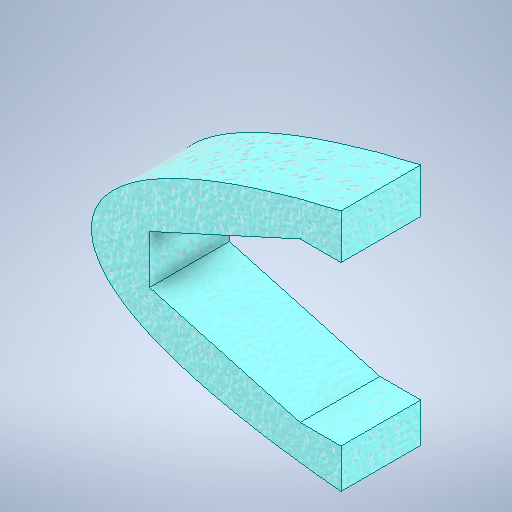
# Autodesk Inventor part: 2414 basic aerofoil
Saved by Autodesk Inventor 2025.1 (Build 291241000, 241)
## iProperties
Created: 2024-11-04
Part Number: 2414 basic aerofoil
Material: Polyurethane Foam
Document SubType Name: Modeling
Designer: johan
Density: 0.032 g/cm^3
Appearance: Coarse Textured - Umber
Author: johan
Autodesk Inventor part; units mm, degrees
ref_plane "YZ Plane" through (0, 0, 0) normal (1, 0, 0) x (0, 1, 0)
ref_plane "XZ Plane" through (0, 0, 0) normal (0, 1, 0) x (-1, 0, 0)
ref_plane "XY Plane" through (0, 0, 0) normal (0, 0, 1) x (1, 0, 0)
sketch "Sketch2" plane through (0, 0, 0) normal (0, 0, 1) x (1, 0, 0)
  spline S0 degree 5 poles (319.65, 0.0573) (319.6503, 0.0612) (319.6024, 0.0717) (319.374, 0.1032) (319.3593, 0.1578) (318.7198, 0.2501) (318.4415, 0.3676) (317.6224, 0.5235) (316.9348, 0.7102) (315.9237, 0.9334) (314.8763, 1.1862) (313.6258, 1.4728) (312.2675, 1.7887) (310.7513, 2.1347) (309.1071, 2.5099) (307.3204, 2.9131) (305.4017, 3.3422) (303.3481, 3.7974) (301.1638, 4.2757) (298.8502, 4.7782) (296.4092, 5.301) (293.8431, 5.8446) (291.1548, 6.4061) (288.3466, 6.9857) (285.4207, 7.5803) (282.3807, 8.1894) (279.2284, 8.8107) (275.968, 9.4437) (272.6016, 10.0865) (269.1329, 10.7361) (265.5656, 11.3942) (261.9019, 12.0551) (258.1469, 12.7207) (254.3029, 13.3883) (250.3742, 14.0555) (246.3647, 14.7217) (242.2776, 15.3854) (238.118, 16.0441) (233.8887, 16.6979) (229.5951, 17.3434) (225.2403, 17.981) (220.8295, 18.6073) (216.3658, 19.2226) (211.8553, 19.8242) (207.3009, 20.4107) (202.7077, 20.9813) (198.0804, 21.5339) (193.4233, 22.0679) (188.7413, 22.58) (184.0389, 23.0713) (179.321, 23.5382) (174.592, 23.982) (169.8567, 24.3971) (165.1201, 24.7874) (160.3872, 25.1472) (155.6604, 25.4776) (150.948, 25.7772) (146.2454, 26.0449) (141.5744, 26.278) (136.9015, 26.4795) (132.2479, 26.6311) (127.6319, 26.7392) (123.054, 26.8) (118.5203, 26.8145) (114.0396, 26.782) (109.6095, 26.702) (105.2515, 26.5748) (100.9335, 26.4032) (96.7486, 26.1785) (92.5169, 25.9219) (88.6332, 25.5912) (84.2398, 25.2771) (81.1881, 24.792) (76.5355, 24.4292) (73.1771, 23.9054) (69.3626, 23.3983) (65.9717, 22.8074) (62.3454, 22.2418) (59.4319, 21.5148) (55.4306, 21.0144) (53.2464, 20.1085) (49.5889, 19.5369) (47.2944, 18.6474) (44.3884, 17.909) (41.914, 17.071) (39.4431, 16.2394) (37.1538, 15.3738) (34.9769, 14.4941) (32.9455, 13.5943) (31.0501, 12.6807) (29.2961, 11.7542) (27.6837, 10.815) (26.2149, 9.8673) (24.8895, 8.9103) (23.7099, 7.9466) (22.6751, 6.976) (21.7869, 6.0003) (21.0459, 5.0186) (20.4526, 4.032) (20.0117, 3.0392) (19.7222, 2.0438) (19.5891, 1.0479) (19.6123, 0.0538) (19.7863, -0.9258) (20.1139, -1.8742) (20.591, -2.7944) (21.2166, -3.6796) (21.9855, -4.5321) (22.8956, -5.3513) (23.9453, -6.1385) (25.1332, -6.8944) (26.4582, -7.6188) (27.9184, -8.3123) (29.5136, -8.9751) (31.2409, -9.6071) (33.0997, -10.2066) (35.0892, -10.7758) (37.2002, -11.3131) (39.4562, -11.8174) (41.7927, -12.2939) (44.3651, -12.7275) (46.7744, -13.1584) (50.0006, -13.4811) (52.1532, -13.8926) (55.9371, -14.1294) (58.2153, -14.4716) (61.732, -14.6854) (64.8012, -14.9153) (68.2287, -15.092) (71.6338, -15.2498) (75.1915, -15.3722) (78.8137, -15.4692) (82.5326, -15.5359) (86.3291, -15.5764) (90.2061, -15.5901) (94.1575, -15.5787) (98.1812, -15.5438) (102.2727, -15.4851) (106.4286, -15.4059) (110.6456, -15.3062) (114.9188, -15.1867) (119.2459, -15.0512) (123.6218, -14.8988) (128.0442, -14.7319) (132.5111, -14.552) (137.0141, -14.3592) (141.5621, -14.1606) (146.1675, -13.9403) (150.787, -13.7052) (155.434, -13.4523) (160.0951, -13.1857) (164.7676, -12.9046) (169.4465, -12.6129) (174.1261, -12.3082) (178.8033, -11.9955) (183.4722, -11.6727) (188.1294, -11.3426) (192.7696, -11.0072) (197.3886, -10.6641) (201.9818, -10.3188) (206.5448, -9.9678) (211.0728, -9.6157) (215.5623, -9.2611) (220.007, -8.9047) (224.4048, -8.5497) (228.7493, -8.193) (233.0373, -7.8393) (237.2647, -7.4865) (241.4259, -7.1353) (245.5189, -6.7884) (249.5374, -6.4441) (253.4791, -6.104) (257.3389, -5.7683) (261.1136, -5.4376) (264.7987, -5.113) (268.3914, -4.7937) (271.8871, -4.4807) (275.2826, -4.1749) (278.5752, -3.8759) (281.7596, -3.585) (284.8354, -3.3021) (287.7962, -3.0278) (290.6419, -2.763) (293.3672, -2.5063) (295.9712, -2.2616) (298.4496, -2.0246) (300.8012, -1.801) (303.0222, -1.5859) (305.1122, -1.3849) (307.0656, -1.194) (308.8864, -1.0166) (310.5623, -0.8504) (312.1091, -0.6993) (313.4946, -0.5587) (314.7717, -0.4371) (315.8416, -0.3205) (316.8735, -0.2329) (317.5785, -0.1363) (318.4116, -0.0907) (318.7022, -0.0102) (319.3489, -0.0035) (319.3702, 0.0486) (319.6008, 0.0494) (319.6497, 0.0535) (319.65, 0.0573) knots 0 0 0 0 0 0 0.001408 0.00264 0.004356 0.006446 0.008836 0.011489 0.014377 0.017481 0.020784 0.024273 0.027936 0.031764 0.035749 0.039881 0.044154 0.048561 0.053096 0.057754 0.062528 0.067414 0.072407 0.077502 0.082694 0.08798 0.093354 0.098813 0.104353 0.10997 0.115661 0.12142 0.127246 0.133133 0.13908 0.145081 0.151134 0.157236 0.163382 0.16957 0.175796 0.182056 0.188349 0.19467 0.201015 0.207383 0.213769 0.220171 0.226584 0.233007 0.239435 0.245866 0.252297 0.258724 0.265143 0.271553 0.277953 0.284342 0.290717 0.297076 0.303415 0.309727 0.316008 0.322252 0.328458 0.334623 0.340742 0.346813 0.352832 0.358737 0.364641 0.370484 0.376262 0.381972 0.38767 0.393237 0.398773 0.404177 0.409526 0.414755 0.419892 0.424884 0.429828 0.434639 0.439375 0.444001 0.448513 0.452908 0.457182 0.461332 0.465356 0.469252 0.473017 0.476652 0.480159 0.483541 0.486805 0.489964 0.493033 0.496034 0.49899 0.501921 0.504852 0.507807 0.510807 0.513874 0.517028 0.520286 0.523658 0.527152 0.530771 0.534517 0.538388 0.542384 0.546503 0.550741 0.555096 0.559563 0.56414 0.568856 0.573641 0.578576 0.583553 0.588622 0.593747 0.59899 0.604262 0.609667 0.615146 0.620698 0.626318 0.632003 0.637751 0.643558 0.649421 0.655338 0.661304 0.667318 0.673375 0.679474 0.685611 0.691783 0.697987 0.704223 0.710491 0.716788 0.723111 0.729457 0.735821 0.742195 0.748577 0.754963 0.761351 0.767737 0.774118 0.780492 0.786854 0.793202 0.799533 0.805843 0.812129 0.818388 0.824617 0.830812 0.836971 0.843089 0.849164 0.855191 0.861169 0.867093 0.872959 0.878764 0.884505 0.890178 0.895779 0.901304 0.906749 0.912111 0.917384 0.922566 0.927651 0.932635 0.937513 0.942281 0.946932 0.951462 0.955865 0.960134 0.964263 0.968244 0.97207 0.975732 0.97922 0.982521 0.985624 0.988512 0.991164 0.993554 0.995644 0.99736 0.998592 1 1 1 1 1 1
  circle A0 centre (80.6499, 4.6494) radius 14
  line L0 (80.6499, 4.6494) -> (80.6499, 24.7974) construction
  circle A1 centre (209.65, 4.6494) radius 4.2
  line L1 (80.6499, 4.6494) -> (209.65, 4.6494) construction
  line L2 (319.65, 0.0573) -> (219.65, 0.0573) construction
  line L3 (219.65, 18.7671) -> (219.65, -8.9327) construction
  line L4 (28.0057, 4.5054) -> (28.0057, -2.4946)
  line L5 (19.6271, 1.0326) -> (319.65, 0.0573) construction
  line L6 (49.7105, 14.4213) -> (55.6079, 14.4213)
  line L7 (49.7105, -8.4915) -> (55.6079, -8.4915)
  line L8 (28.0057, 4.5054) -> (49.7105, 14.4213)
  line L9 (28.0057, -2.4946) -> (49.7105, -8.4915)
  line L10 (55.6079, 14.4213) -> (55.6079, 20.8726)
  line L11 (55.6079, -8.4915) -> (55.6079, -14.1513)
  point P0 (0, 0)
  point P1 (319.3571, 0.1272)
  point P2 (318.9917, 0.2142)
  point P3 (318.4802, 0.3354)
  point P4 (317.8238, 0.4911)
  point P5 (317.0222, 0.6801)
  point P6 (316.0769, 0.9024)
  point P7 (314.9885, 1.1568)
  point P8 (313.7582, 1.443)
  point P9 (312.3866, 1.7598)
  point P10 (310.8752, 2.1063)
  point P11 (309.2258, 2.4819)
  point P12 (307.4393, 2.8854)
  point P13 (305.5178, 3.3153)
  point P14 (303.4628, 3.7707)
  point P15 (301.2764, 4.2501)
  point P16 (298.9607, 4.7526)
  point P17 (296.5175, 5.2764)
  point P18 (293.9492, 5.8203)
  point P19 (291.2585, 6.3828)
  point P20 (288.4478, 6.9627)
  point P21 (285.5195, 7.5582)
  point P22 (282.4766, 8.1678)
  point P23 (279.3218, 8.79)
  point P24 (276.0584, 9.4236)
  point P25 (272.6891, 10.0668)
  point P26 (269.2175, 10.7178)
  point P27 (265.6469, 11.3757)
  point P28 (261.9803, 12.0381)
  point P29 (258.2219, 12.7041)
  point P30 (254.3747, 13.3722)
  point P31 (250.4426, 14.0403)
  point P32 (246.4295, 14.7072)
  point P33 (242.339, 15.3714)
  point P34 (238.1756, 16.0311)
  point P35 (233.9429, 16.6851)
  point P36 (229.6454, 17.3316)
  point P37 (225.287, 17.9694)
  point P38 (220.8722, 18.5967)
  point P39 (216.4049, 19.2123)
  point P40 (211.8902, 19.8144)
  point P41 (207.332, 20.4015)
  point P42 (202.7348, 20.9724)
  point P43 (198.1034, 21.5256)
  point P44 (193.4423, 22.0596)
  point P45 (188.7563, 22.5726)
  point P46 (184.0499, 23.0637)
  point P47 (179.3279, 23.5314)
  point P48 (174.5948, 23.9745)
  point P49 (169.8554, 24.3909)
  point P50 (165.1148, 24.7803)
  point P51 (160.3775, 25.1406)
  point P52 (155.648, 25.4709)
  point P53 (150.9317, 25.7703)
  point P54 (146.2331, 26.0373)
  point P55 (141.557, 26.2707)
  point P56 (136.8821, 26.4681)
  point P57 (132.221, 26.6211)
  point P58 (127.5965, 26.7282)
  point P59 (123.0134, 26.7888)
  point P60 (118.4762, 26.8026)
  point P61 (113.9903, 26.7693)
  point P62 (109.5602, 26.6886)
  point P63 (105.191, 26.5611)
  point P64 (100.8866, 26.3865)
  point P65 (96.6524, 26.1648)
  point P66 (92.4926, 25.8972)
  point P67 (88.4117, 25.5837)
  point P68 (84.4142, 25.2255)
  point P69 (80.8999, 24.8247)
  point P70 (76.6859, 24.3774)
  point P71 (72.9632, 23.8899)
  point P72 (69.3401, 23.3613)
  point P73 (65.8208, 22.7937)
  point P74 (62.4086, 22.1883)
  point P75 (59.1071, 21.5463)
  point P76 (52.8494, 20.1606)
  point P77 (49.7105, 19.4213)
  point P78 (47.0738, 18.6507)
  point P79 (44.3741, 17.8542)
  point P80 (41.8034, 17.0322)
  point P81 (39.3638, 16.1874)
  point P82 (37.0583, 15.3213)
  point P83 (34.8884, 14.4363)
  point P84 (32.8568, 13.5339)
  point P85 (30.965, 12.6165)
  point P86 (29.2145, 11.6859)
  point P87 (27.6071, 10.7436)
  point P88 (26.1443, 9.792)
  point P89 (24.827, 8.8323)
  point P90 (23.6567, 7.8663)
  point P91 (22.6337, 6.8952)
  point P92 (21.7592, 5.9208)
  point P93 (21.0335, 4.944)
  point P94 (20.4572, 3.966)
  point P95 (20.0309, 2.9874)
  point P96 (19.754, 2.0097)
  point P97 (19.6499, 0.0573)
  point P98 (19.8206, -0.9033)
  point P99 (20.1377, -1.8357)
  point P100 (20.6003, -2.7402)
  point P101 (21.2081, -3.6159)
  point P102 (21.9599, -4.4628)
  point P103 (22.8545, -5.2806)
  point P104 (23.891, -6.069)
  point P105 (25.0682, -6.8277)
  point P106 (26.3846, -7.5561)
  point P107 (27.8384, -8.2539)
  point P108 (29.4284, -8.9211)
  point P109 (31.1522, -9.5571)
  point P110 (33.0086, -10.1613)
  point P111 (34.9949, -10.734)
  point P112 (37.1093, -11.2746)
  point P113 (39.3497, -11.7828)
  point P114 (41.7134, -12.2586)
  point P115 (44.198, -12.702)
  point P116 (46.8014, -13.1127)
  point P117 (49.7105, -13.4915)
  point P118 (52.3532, -13.8357)
  point P119 (58.3469, -14.4294)
  point P120 (61.5023, -14.6781)
  point P121 (64.7591, -14.8953)
  point P122 (68.1149, -15.0813)
  point P123 (71.5661, -15.237)
  point P124 (75.1094, -15.3627)
  point P125 (78.7418, -15.4596)
  point P126 (82.46, -15.528)
  point P127 (86.2607, -15.5691)
  point P128 (90.14, -15.5838)
  point P129 (94.0946, -15.5733)
  point P130 (98.1212, -15.5388)
  point P131 (102.2159, -15.4812)
  point P132 (106.3751, -15.4023)
  point P133 (110.5952, -15.303)
  point P134 (114.872, -15.1845)
  point P135 (119.2022, -15.0489)
  point P136 (123.5813, -14.8971)
  point P137 (128.006, -14.7306)
  point P138 (132.4718, -14.5509)
  point P139 (136.9748, -14.3598)
  point P140 (141.5285, -14.1576)
  point P141 (146.1365, -13.9383)
  point P142 (150.7679, -13.7022)
  point P143 (155.4191, -13.4499)
  point P144 (160.0853, -13.1829)
  point P145 (164.7617, -12.9024)
  point P146 (169.4444, -12.6099)
  point P147 (174.1283, -12.306)
  point P148 (178.8092, -11.9925)
  point P149 (183.4823, -11.67)
  point P150 (188.1434, -11.34)
  point P151 (192.7877, -11.0037)
  point P152 (197.4107, -10.6614)
  point P153 (202.0079, -10.3149)
  point P154 (206.5748, -9.9645)
  point P155 (211.1069, -9.6117)
  point P156 (215.6, -9.2568)
  point P157 (220.049, -8.9007)
  point P158 (224.4503, -8.5446)
  point P159 (228.7988, -8.1885)
  point P160 (233.0906, -7.8339)
  point P161 (237.3215, -7.4808)
  point P162 (241.4867, -7.1298)
  point P163 (245.5829, -6.7821)
  point P164 (249.6053, -6.4377)
  point P165 (253.5503, -6.0972)
  point P166 (257.4137, -5.7612)
  point P167 (261.1916, -5.4303)
  point P168 (264.8801, -5.1051)
  point P169 (268.4759, -4.7856)
  point P170 (271.9748, -4.4724)
  point P171 (275.3735, -4.1661)
  point P172 (278.6687, -3.867)
  point P173 (281.8565, -3.5757)
  point P174 (284.9345, -3.2925)
  point P175 (287.8985, -3.018)
  point P176 (290.7464, -2.7525)
  point P177 (293.4746, -2.4963)
  point P178 (296.0807, -2.2503)
  point P179 (298.5617, -2.0142)
  point P180 (300.9152, -1.7892)
  point P181 (303.1388, -1.575)
  point P182 (305.2301, -1.3728)
  point P183 (307.1867, -1.1823)
  point P184 (309.0071, -1.0041)
  point P185 (310.6886, -0.8385)
  point P186 (312.2303, -0.6861)
  point P187 (313.6298, -0.5472)
  point P188 (314.8862, -0.4221)
  point P189 (315.9977, -0.3108)
  point P190 (316.9637, -0.2139)
  point P191 (317.7827, -0.1314)
  point P192 (318.4538, -0.0636)
  point P193 (318.9767, -0.0108)
  point P194 (319.3505, 0.027)
  point P195 (319.5749, 0.0498)
  point P196 (28.0057, 1.0054)
  dimension "d2" = 300.0001
  dimension "d9" = 28
  dimension "d15" = 61
  dimension "d16" = 20.148
  dimension "d18" = 8.4
  dimension "d19" = 110
  dimension "d22" = 100
  dimension "d23" = 7
  dimension "d24" = 5
  dimension "d25" = 5
  constraints: 24 end point, 4 vertical, 2 centre point, 2 horizontal, 1 collinear, 1 midpoint, 1 point on line, 203 other
  measures "d2" distance of L2.start point (19.65, 0.057)
  measures "d9" diameter of A0
  measures "d15" horizontal distance of point (19.65, 0.057) L0.start
  measures "d16" distance of L0.start L0.end
  measures "d18" diameter of A1
  measures "d19" horizontal distance of L2.start L1.end
  measures "d22" distance of L2.start L2.end
  measures "d23" distance of L4.start L4.end
  measures "d24" distance from line of point (49.71, 19.421) L6
  measures "d25" distance from line of point (49.71, -13.491) L7
extrude "Extrusion5" add sketch "Sketch2" along normal blind 11.5 contours L10 L6 L8 L4 L9 L7 L11 S0 picked at (37.3485, 11.0408)
body "Solid5"
